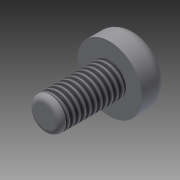
# Autodesk Inventor part: M3x6
Saved by Autodesk Inventor 2015 (Build 190159000, 159)
## iProperties
Created: 2015-06-15
Part Number: M3x6
Material: Generic
Document SubType Name: Modeling
Designer: Jufo
Density: 1 g/cm^3
Appearance: Default
Author: Jufo
Autodesk Inventor part; units mm, degrees
ref_plane "YZ Plane" through (0, 0, 0) normal (1, 0, 0) x (0, 1, 0)
ref_plane "XZ Plane" through (0, 0, 0) normal (0, 1, 0) x (-1, 0, 0)
ref_plane "XY Plane" through (0, 0, 0) normal (0, 0, 1) x (1, 0, 0)
sketch "Sketch1" plane through (0, 0, 0) normal (0, 1, 0) x (-1, 0, 0)
  circle A0 centre (0, 0) radius 1.5
  dimension "d0" = 3
  constraints: 1 centre point, 1 coincident
  measures "d0" diameter of A0
extrude "Extrusion1" add sketch "Sketch1" along normal blind 6
sketch "Sketch2" plane through (0, 6, 0) normal (0, 1, 0) x (1, 0, 0)
  circle A0 centre (0, 0) radius 1.5 projected
  circle A1 centre (0, 0) radius 3
  dimension "d3" = 6
  constraints: 1 centre point, 1 coincident
  measures "d3" diameter of A1
extrude "Extrusion2" add sketch "Sketch2" along normal blind 2.4 contours A0 | A1
fillet "Fillet4" radius 0.5 1 edges at (1.5, 0, 0)
thread "Thread2" size "M3x0.5" class "6g" standard "ANSI Metric M Profile" full length
fillet "Fillet5" radius 1 1 edges at (-3, 8.4, 0)
sketch "Sketch5" plane through (0, 8.4, 0) normal (0, 1, 0) x (1, 0, 0)
  circle A0 centre (0, 0) radius 2 projected
  line L0 (-0.3, 0) -> (-0.3, 1.9774)
  line L1 (0.3, 1.9774) -> (0.3, -1.9774)
  line L2 (-0.3, 1.9774) -> (-0.3, -1.9774)
  line L3 (0, 0.3) -> (-1.9774, 0.3)
  line L4 (-1.9774, 0.3) -> (1.9774, 0.3)
  line L5 (-1.9774, -0.3) -> (1.9774, -0.3)
  dimension "d32" = 0.3
  dimension "d33" = 0.3
  dimension "d35" = 0.3
  dimension "d36" = 0.3
  constraints: 12 end point, 2 parallel, 2 perpendicular, 1 point on line, 1 vertical, 9 other
  measures "d32" distance from line of point (0, 0) L4
  measures "d33" distance from line of point (0, 0) L5
  measures "d35" distance from line of L1 point (0, 0)
  measures "d36" distance from line of L0 point (0, 0)
extrude "Extrusion4" cut sketch "Sketch5" against normal blind 1 contours A0 L5 L1 L4 | L1 L4 L3 L0 A0 | L1 L5 L2 L0 L3 L4 | A0 L2 L5 L1 | L5 A0 L3 L0 L2
body "Solid1"
